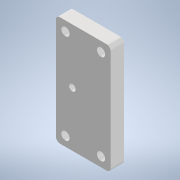
# Autodesk Inventor part: 10_Mountinplate_Mirrors_v0
Saved by Autodesk Inventor 2022 (Build 260153000, 153)
## iProperties
Created: 2022-05-18
Part Number: 10_Mountinplate_Mirrors_v0
Material: Generisch
Document SubType Name: Modeling
Designer: diederichbenedict
Density: 1 g/cm^3
Appearance: Vorgabe
Author: diederichbenedict
Autodesk Inventor part; units mm, degrees
ref_plane "YZ Plane" through (0, 0, 0) normal (1, 0, 0) x (0, 1, 0)
ref_plane "XZ Plane" through (0, 0, 0) normal (0, 1, 0) x (-1, 0, 0)
ref_plane "XY Plane" through (0, 0, 0) normal (0, 0, 1) x (1, 0, 0)
ref_plane "Arbeitsebene1" through (0, 0, 0) normal (0, 0, 1) x (1, 0, 0)
sketch "Skizze1" plane through (0, 0, 0) normal (0, 0, 1) x (1, 0, 0)
  line L0 (0.635, 25.527) -> (10.16, 25.527) projected
  line L1 (0.635, 25.527) -> (0.635, 0) projected
  line L2 (0.635, 0) -> (10.16, 0) projected
  line L3 (10.16, 0) -> (10.16, 25.527) projected
  line L4 (30.08, -27.3) -> (-3.92, -27.3)
  line L5 (-6.92, -24.3) -> (-6.92, 49.7)
  line L6 (-3.92, 52.7) -> (30.08, 52.7)
  line L7 (33.08, -27.3) -> (-6.92, 52.7) construction
  line L8 (-6.92, -27.3) -> (33.08, 52.7) construction
  arc A0 (30.08, -27.3) -> (33.08, -24.3) centre (30.08, -24.3) ccw
  arc A1 (-6.92, -24.3) -> (-3.92, -27.3) centre (-3.92, -24.3) ccw
  arc A2 (-3.92, 52.7) -> (-6.92, 49.7) centre (-3.92, 49.7) ccw
  arc A3 (33.08, 49.7) -> (30.08, 52.7) centre (30.08, 49.7) ccw
  circle A4 centre (5.08, 12.7) radius 2.3813
  line L9 (33.08, -24.3) -> (33.08, 49.7)
  point P0 (0, 0)
  point P1 (13.08, 12.7)
  dimension "d1" = 80
  dimension "d2" = 3
  dimension "d7" = 0
  dimension "d8" = 8
  constraints: 12 end point, 8 point on circle, 7 tangent, 6 point on line, 5 centre point, 3 equal radius, 1 horizontal, 1 midpoint, 1 parallel, 1 perpendicular, 1 vertical, 2 other
  measures "d1" distance of L8.start L7.end
  measures "d2" radius of A0
  measures "d7" vertical distance of A4.centre point (13.08, 12.7)
  measures "d8" distance of point (13.08, 12.7) A4.centre
ref_plane "Arbeitsebene2" through (291.5074, -13.3966, 8.6065) normal (0, 0, 1) x (0.898794, -0.4383711, 0)
extrude "Extrusion1" add sketch "Skizze1" along normal up to surface (8.6065 mm away) contours L0 L3 L2 L1 | L4 A1 L5 A2 L6 A3 L9 A0
sketch "Skizze3" plane through (0, 0, 0) normal (0, 0, -1) x (-1, 0, 0)
  arc A0 (-30.08, 52.7) -> (-33.08, 49.7) centre (-30.08, 49.7) ccw projected
  line L0 (-33.08, -24.3) -> (-33.08, 49.7) projected
  arc A1 (-33.08, -24.3) -> (-30.08, -27.3) centre (-30.08, -24.3) ccw projected
  line L1 (3.92, -27.3) -> (-30.08, -27.3) projected
  arc A2 (3.92, -27.3) -> (6.92, -24.3) centre (3.92, -24.3) ccw projected
  line L2 (6.92, 49.7) -> (6.92, -24.3) projected
  arc A3 (6.92, 49.7) -> (3.92, 52.7) centre (3.92, 49.7) ccw projected
  line L3 (-30.08, 52.7) -> (3.92, 52.7) projected
  circle A4 centre (-5.08, 12.7) radius 2.3813 projected
  line L4 (-26.08, 45.7) -> (-0.08, 45.7)
  line L5 (-0.08, 45.7) -> (-0.08, -20.3)
  line L6 (-0.08, -20.3) -> (-26.08, -20.3)
  line L7 (-26.08, -20.3) -> (-26.08, 45.7)
  point P0 (0, 0)
  dimension "d9" = 7
  constraints: 8 end point, 3 other
  measures "d9" distance between parallel lines of L0 L7
hole "Bohrung1" at (26.08, 45.7, 0) at (26.08, -20.3, 0) at (0.08, -20.3, 0) at (0.08, 45.7, 0) direction (0, 0, 1) diameter 8 depth 8 tip angle 118
sketch "Skizze4" plane through (-6.92, -24.3, 0) normal (-1, 0, 0) x (0, 0, 1)
  circle A0 centre (-6.731, 17.95) radius 7.366 projected
  circle A1 centre (-6.731, 17.95) radius 9.366
  circle A2 centre (-6.731, 56.05) radius 7.366
  circle A3 centre (-6.731, 56.05) radius 9.366
  point P0 (0, 24.3)
  dimension "d17" = 2
  constraints: 3 centre point, 1 equal radius, 2 other
  measures "d17" radial gap between concentric circles of A0 A1
ref_plane "Arbeitsebene3" through (0, -11.176, -49.276) normal (-1, 0, 0) x (0, 0.0000004, 1)
extrude "Extrusion2" cut sketch "Skizze4" against normal up to surface (6.92 mm away) contours A0 | A1 | A2 | A3
sketch "Skizze5" plane through (0, 0, 0) normal (0, 0, -1) x (-1, 0, 0)
  circle A0 centre (-5.08, 12.7) radius 2.3813 projected
  line L0 (6.92, -12.8627) -> (0, -12.8627) projected
  line L1 (0, -12.8627) -> (0, 0.1627) projected
  line L2 (0, 0.1627) -> (6.92, 0.1627) projected
  line L3 (6.92, 49.7) -> (6.92, 38.2627) projected
  arc A1 (6.92, 49.7) -> (3.92, 52.7) centre (3.92, 49.7) ccw projected
  line L4 (-30.08, 52.7) -> (3.92, 52.7) projected
  arc A2 (-30.08, 52.7) -> (-33.08, 49.7) centre (-30.08, 49.7) ccw projected
  line L5 (-33.08, -24.3) -> (-33.08, 49.7) projected
  arc A3 (-33.08, -24.3) -> (-30.08, -27.3) centre (-30.08, -24.3) ccw projected
  line L6 (3.92, -27.3) -> (-30.08, -27.3) projected
  arc A4 (3.92, -27.3) -> (6.92, -24.3) centre (3.92, -24.3) ccw projected
  line L7 (6.92, -12.8627) -> (6.92, -24.3) projected
  circle A5 centre (-0.08, 45.7) radius 4 projected
  circle A6 centre (-26.08, -20.3) radius 4 projected
  circle A7 centre (-26.08, 45.7) radius 4 projected
  circle A8 centre (-0.08, -20.3) radius 4 projected
  line L8 (-0.635, 29.1338) -> (-10.16, 29.1338) projected
  line L9 (-0.635, -2.2814) -> (-10.16, -2.2814) projected
  line L10 (-10.16, -2.2814) -> (-10.16, 29.1338)
  line L11 (-0.635, 29.1338) -> (-0.635, -2.2814)
  line L12 (0, 0.1627) -> (0, -12.8627) projected
  line L13 (-10.36, 29.3338) -> (-0.435, 29.3338)
  line L14 (-0.435, 29.3338) -> (-0.435, -2.4814)
  line L15 (-0.435, -2.4814) -> (-10.36, -2.4814)
  line L16 (-10.36, -2.4814) -> (-10.36, 29.3338)
  line L17 (6.92, 25.2373) -> (6.92, 0.1627) projected
  line L18 (6.92, 25.2373) -> (0, 25.2373) projected
  line L19 (0, 25.2373) -> (0, 38.2627) projected
  line L20 (0, 38.2627) -> (6.92, 38.2627) projected
  point P0 (0, 0)
  dimension "d20" = 0.2
  constraints: 12 end point, 1 parallel, 1 vertical, 3 other
  measures "d20" distance between parallel lines of L11 L14
ref_plane "Arbeitsebene4" through (-0.1034, 27.5049, -1.27) normal (0, 0.0000004, 1) x (1, 0, 0)
extrude "Extrusion3" add sketch "Skizze5" along normal up to surface (1.27 mm away) contours L7 A4 L6 A3 L5 A2 L4 A1 L3 L20 L19 L18 L17 L2 L1 L0
